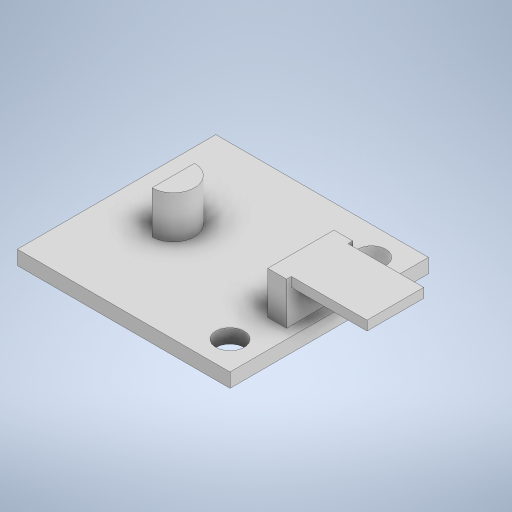
# Autodesk Inventor part: DS18B20
Saved by Autodesk Inventor 2024 (Build 280153000, 153)
## iProperties
Created: 2025-03-12
Part Number: DS18B20
Material: Generic
Document SubType Name: Modeling
Designer: 5454s
Density: 1 g/cm^3
Appearance: Default
Author: 5454s
Autodesk Inventor part; units mm, degrees
ref_plane "YZ Plane" through (0, 0, 0) normal (1, 0, 0) x (0, 1, 0)
ref_plane "XZ Plane" through (0, 0, 0) normal (0, 1, 0) x (-1, 0, 0)
ref_plane "XY Plane" through (0, 0, 0) normal (0, 0, 1) x (1, 0, 0)
sketch "Sketch1" plane through (0, 0, 0) normal (0, 1, 0) x (-1, 0, 0)
  line L0 (0, 0) -> (22.5, 0)
  line L1 (22.5, 0) -> (22.5, -21)
  line L2 (22.5, -21) -> (0, -21)
  line L3 (0, -21) -> (0, 0)
  circle A0 centre (3, -3) radius 1.5
  circle A1 centre (3, -18) radius 1.5
  line L4 (22.5, -10.5) -> (0, -10.5)
  dimension "d0" = 21
  dimension "d1" = 22.5
  dimension "d2" = 3
  dimension "d5" = 3
  dimension "d8" = 3
  dimension "d25" = 15
  dimension "d26" = 3
  constraints: 10 end point, 2 centre point, 2 midpoint, 2 parallel, 1 equal radius, 1 horizontal, 1 perpendicular
  measures "d0" distance of L2.end L0.start
  measures "d1" distance of L1.end L2.end
  measures "d2" diameter of A0
  measures "d5" distance from line of L3 A1.centre
  measures "d8" distance from line of L3 A0.centre
  measures "d25" distance of A0.centre A1.centre
  measures "d26" distance from line of L2 A1.centre
extrude "Extrusion1" add sketch "Sketch1" along normal blind 1.5
sketch "Sketch2" plane through (0, 1.5, 0) normal (0, 1, 0) x (1, 0, 0)
  line L0 (-3, 7) -> (-1, 7)
  line L1 (-1, 7) -> (-1, 14)
  line L2 (-1, 14) -> (-3, 14)
  line L3 (-3, 14) -> (-3, 7)
  line L4 (-16.5, 8.25) -> (-16.5, 12.75)
  circle A0 centre (-16.5, 10.5) radius 2.25
  line L5 (-22.5, 21) -> (-22.5, 0) projected
  line L6 (-22.5, 10.5) -> (0, 10.5)
  line L7 (0, 0) -> (0, 21) projected
  dimension "d11" = 4.5
  dimension "d12" = 7
  dimension "d13" = 2
  dimension "d14" = 1
  dimension "d15" = 6
  constraints: 12 end point, 3 midpoint, 2 parallel, 1 horizontal, 1 perpendicular, 1 point on line, 1 vertical, 4 other
  measures "d12" distance of L0.end L1.end
  measures "d13" distance of L0.start L0.end
  measures "d14" distance between parallel lines of L7 L1
  measures "d15" distance between parallel lines of L5 L4
extrude "Extrusion2" add sketch "Sketch2" along normal blind 4.5 contours L3 L6 L1 L0 | A0 L4 L6 | L6 L4 A0 | L3 L2 L1 L6 picked at (-15.2379, 9.707) picked at (-15.707, 11.7621)
sketch "Sketch3" plane through (-1, 1.5, -7) normal (1, 0, 0) x (0, 0, -1)
  line L0 (0.5, 3.5) -> (6.5, 3.5)
  line L1 (6.5, 3.5) -> (6.5, 4.5)
  line L2 (6.5, 4.5) -> (0.5, 4.5)
  line L3 (0.5, 4.5) -> (0.5, 3.5)
  line L4 (-7, 0) -> (14, 0) projected
  line L5 (0, 4.5) -> (7, 4.5) projected
  line L6 (0, 0) -> (0, 4.5) projected
  line L7 (7, 0) -> (7, 4.5) projected
  point P0 (-7, -1.5)
  point P1 (0.5, 4)
  dimension "d18" = 6
  dimension "d19" = 1
  dimension "d21" = 0.5
  dimension "d22" = 0.5
  constraints: 8 end point, 2 parallel, 1 collinear, 1 horizontal, 1 midpoint, 1 perpendicular
  measures "d18" distance of L0.start L0.end
  measures "d19" distance of L2.end L0.start
  measures "d21" distance from line of L6 point (0.5, 4)
  measures "d22" distance from line of L7 L0.end
extrude "Extrusion3" add sketch "Sketch3" along normal blind 8 contours L3 L2 L1 L0
body "Solid1"
